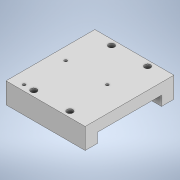
# Autodesk Inventor part: P132SupportCamera
Saved by Autodesk Inventor 2020 (Build 240168000, 168)
## iProperties
Created: 2021-07-29
Part Number: P132SupportCamera
Material: Generic
Document SubType Name: Modeling
Designer: brice.dubuis
Density: 1 g/cm^3
Appearance: Default
Author: brice.dubuis
Autodesk Inventor part; units mm, degrees
ref_plane "YZ Plane" through (0, 0, 0) normal (1, 0, 0) x (0, 1, 0)
ref_plane "XZ Plane" through (0, 0, 0) normal (0, 1, 0) x (-1, 0, 0)
ref_plane "XY Plane" through (0, 0, 0) normal (0, 0, 1) x (1, 0, 0)
sketch "Sketch1" plane through (0, 0, 0) normal (0, 1, 0) x (-1, 0, 0)
  line L0 (0, 0) -> (57, 0)
  line L1 (57, 0) -> (57, -64)
  line L2 (57, -64) -> (0, -64)
  line L3 (0, -64) -> (0, 0)
  dimension "d0" = 57
  dimension "d1" = 64
  constraints: 8 end point, 2 parallel, 1 horizontal, 1 perpendicular
  measures "d0" distance between parallel lines of L3 L1
  measures "d1" distance between parallel lines of L0 L2
extrude "Extrusion1" add sketch "Sketch1" along normal blind 8
sketch "Sketch2" plane through (0, 8, 0) normal (0, 1, 0) x (1, 0, 0)
  line L0 (-57, 64) -> (-57, 0) projected
  line L1 (-57, 0) -> (0, 0) projected
  line L2 (0, 64) -> (-57, 64) projected
  point P0 (-41, 4)
  point P1 (-15, 4)
  point P2 (-41, 60)
  point P3 (-15, 60)
  dimension "d4" = 26
  dimension "d5" = 16
  dimension "d6" = 4
  dimension "d7" = 4
  dimension "d8" = 4
  dimension "d9" = 4
  dimension "d10" = 26
  dimension "d11" = 16
  measures "d4" distance of point (-15, 4) point (-41, 4)
  measures "d5" distance from line of L0 point (-41, 4)
  measures "d6" distance from line of L1 point (-41, 4)
  measures "d7" distance from line of L1 point (-15, 4)
  measures "d8" distance from line of L2 point (-41, 60)
  measures "d9" distance from line of L2 point (-15, 60)
  measures "d10" distance of point (-41, 60) point (-15, 60)
  measures "d11" distance from line of L0 point (-41, 60)
sketch "Sketch3" plane through (0, 0, 0) normal (0, -1, 0) x (1, 0, 0)
  line L0 (0, -64) -> (-57, -64) projected
  line L1 (0, 0) -> (0, -64) projected
  line L2 (-57, -64) -> (0, -64)
  line L3 (0, -64) -> (0, -55)
  line L4 (0, -55) -> (-57, -55)
  line L5 (-57, -55) -> (-57, -64)
  line L6 (-57, -64) -> (-57, 0) projected
  line L7 (-57, 0) -> (0, 0)
  line L8 (0, 0) -> (0, -9)
  line L9 (0, -9) -> (-57, -9)
  line L10 (-57, -9) -> (-57, 0)
  dimension "d12" = 9
  dimension "d13" = 9
  constraints: 16 end point, 4 parallel, 2 horizontal, 2 perpendicular, 2 point on line
  measures "d12" distance between parallel lines of L0 L4
  measures "d13" distance between parallel lines of L7 L9
extrude "Extrusion2" add sketch "Sketch3" along normal blind 7 contours L0 L5 L4 L1 | L9 L6 L7 L1
hole "Hole1" at (-41, 8, -4) at (-15, 8, -4) at (-41, 8, -60) at (-15, 8, -60) direction (0, -1, 0) diameter 4.3 end through all
sketch "Sketch4" plane through (0, 8, 0) normal (0, 1, 0) x (1, 0, 0)
  line L0 (-57, 0) -> (0, 0) projected
  line L1 (-57, 64) -> (-57, 0) projected
  line L2 (0, 0) -> (0, 64) projected
  line L3 (-63.6235, 34) -> (1.4941, 34) construction
  line L4 (-48, -4.864) -> (-48, 68.9429) construction
  point P0 (-48, 4)
  point P1 (-48, 34)
  point P2 (-18, 34)
  dimension "d28" = 4
  dimension "d30" = 9
  dimension "d41" = 30
  dimension "d42" = 30
  constraints: 4 end point, 4 point on line, 1 horizontal, 1 vertical
  measures "d28" distance from line of L0 point (-48, 4)
  measures "d30" distance from line of L1 point (-48, 34)
  measures "d41" distance from line of point (-18, 34) L4
  measures "d42" distance from line of point (-48, 4) L3
hole "Hole2" at (-48, 8, -4) at (-48, 8, -34) at (-18, 8, -34) direction (0, -1, 0) diameter 2.05 end through all
body "Solid1"
